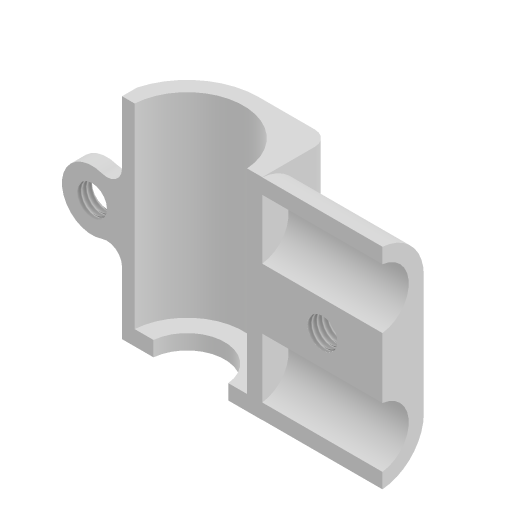
# Autodesk Inventor part: LinearBearingHolderThreaded
Saved by Autodesk Inventor 2023 (Build 270158000, 158)
## iProperties
Created: 2022-10-31
Part Number: LinearBearingHolderThreaded
Material: Generic
Document SubType Name: Modeling
Designer: deli
Density: 1 g/cm^3
Appearance: Default
Author: deli
Autodesk Inventor part; units mm, degrees
ref_plane "YZ Plane" through (0, 0, 0) normal (1, 0, 0) x (0, 1, 0)
ref_plane "XZ Plane" through (0, 0, 0) normal (0, 1, 0) x (-1, 0, 0)
ref_plane "XY Plane" through (0, 0, 0) normal (0, 0, 1) x (1, 0, 0)
sketch "Sketch2" plane through (0, 0, 0) normal (0, 1, 0) x (-1, 0, 0)
  arc A0 (14.7581, -138.6871) -> (29.7247, -138.6871) centre (22.2414, -138.1871) ccw
  line L0 (12.7414, -138.6871) -> (12.7414, -147.6871)
  arc A1 (22.2414, -147.6871) -> (31.4065, -140.6871) centre (22.2414, -138.1871) ccw
  line L1 (12.7414, -138.6871) -> (14.7581, -138.6871)
  line L2 (34.8429, -138.6871) -> (29.7247, -138.6871)
  line L3 (34.8429, -138.6871) -> (39.4065, -138.6871)
  line L4 (39.4065, -138.6871) -> (39.4065, -140.6871)
  line L5 (39.4065, -140.6871) -> (31.4065, -140.6871)
  line L6 (22.2414, -147.6871) -> (12.7414, -147.6871)
  point P0 (0, 0)
  point P1 (13.7497, -138.6871)
  dimension "d0" = 15
  dimension "d1" = 2
  dimension "d2" = 2
  dimension "d3" = 8
  dimension "d17" = 0.5
  constraints: 14 end point, 4 horizontal, 4 point on circle, 2 centre point, 2 perpendicular, 2 tangent, 1 coincident, 1 collinear, 1 midpoint, 1 vertical
  measures "d0" diameter of A0
  measures "d1" radial gap between concentric circles of A1 A0
  measures "d2" distance of L3.end L4.end
  measures "d3" distance of L4.end L5.end
  measures "d17" vertical distance of A0.centre point (13.75, -138.687)
extrude "Extrusion1" add sketch "Sketch2" along normal blind 26
sketch "Sketch3" plane through (0, 0, 0) normal (0, -1, 0) x (1, 0, 0)
  arc A0 (-31.4065, -140.6871) -> (-22.2414, -147.6871) centre (-22.2414, -138.1871) ccw projected
  line L0 (-12.7414, -147.6871) -> (-22.2414, -147.6871) projected
  line L1 (-12.7414, -138.6871) -> (-12.7414, -147.6871) projected
  line L2 (-39.4065, -140.6871) -> (-39.4065, -138.6871) projected
  line L3 (-31.4065, -140.6871) -> (-39.4065, -140.6871) projected
  line L4 (-39.4065, -138.6871) -> (-29.7247, -138.6871) projected
  arc A1 (-27.2163, -138.6871) -> (-17.2665, -138.6871) centre (-22.2414, -138.1871) ccw
  line L5 (-29.7247, -138.6871) -> (-27.2163, -138.6871)
  line L6 (-17.2665, -138.6871) -> (-12.7414, -138.6871)
  arc A2 (-29.7247, -138.6871) -> (-14.7581, -138.6871) centre (-22.2414, -138.1871) ccw construction
  point P0 (0, 0)
  dimension "d6" = 10
  constraints: 4 end point, 2 collinear, 2 point on circle, 1 centre point, 1 concentric, 1 horizontal, 1 point on line
  measures "d6" diameter of A1
extrude "Extrusion2" add sketch "Sketch3" along normal blind 2
sketch "Sketch5" plane through (-12.7414, -2, -138.6871) normal (1, 0, 0) x (0, 0, -1)
  arc A0 (0, 18.0314) -> (0, 25.9686) centre (-0.5, 22) ccw
  arc A1 (0, 2.0314) -> (0, 9.9686) centre (-0.5, 6) ccw
  arc A2 (5.5, 22) -> (0, 27.9791) centre (-0.5, 22) ccw
  arc A3 (0, 0.0209) -> (5.5, 6) centre (-0.5, 6) ccw
  line L0 (0, 28) -> (9, 28) projected
  line L1 (9, 0) -> (0, 0) projected
  line L2 (0, 0) -> (0, 28) projected
  line L3 (5.5, 22) -> (5.5, 6)
  point P0 (-138.6871, 2)
  point P1 (0, 9.9686)
  point P2 (0, 2.0314)
  point P3 (3.9152, 26)
  dimension "d18" = 8
  dimension "d19" = 2
  dimension "d20" = 0.5
  dimension "d21" = 0.5
  constraints: 8 point on circle, 6 point on line, 4 centre point, 2 coincident, 2 end point, 2 equal radius, 2 tangent, 1 vertical
  measures "d18" diameter of A0
  measures "d19" radial gap between concentric circles of A2 A0
  measures "d20" distance from line of L2 A0.centre
  measures "d21" distance from line of L2 A1.centre
extrude "Extrusion4" add sketch "Sketch5" along normal blind 16 contours A0 L2 A2 L3 A3 A1
sketch "Sketch6" plane through (-39.4065, 26, -138.6871) normal (0, 0, 1) x (1, 0, 0)
  circle A0 centre (4, -14) radius 2
  circle A1 centre (34.6652, -13.9791) radius 2
  line L0 (0, -28) -> (0, 0) projected
  line L1 (12.1902, -28) -> (0, -28) projected
  line L2 (26.6652, -27.9791) -> (42.6652, -27.9791) projected
  line L3 (26.6652, -28) -> (26.6652, 0) projected
  line L4 (42.6652, -25.9686) -> (42.6652, -27.9791) projected
  circle A2 centre (4, -14) radius 4
  line L5 (8, 1.0253) -> (8, -28)
  line L6 (0, 0) -> (9.6818, 0) projected
  arc A3 (8, -19.6569) -> (5.3333, -17.7712) centre (6, -19.6569) ccw
  arc A4 (5.3333, -10.2288) -> (8, -8.3431) centre (6, -8.3431) ccw
  point P0 (39.4065, -26)
  point P1 (26.6652, -9.9686)
  point P2 (26.6652, -2.0314)
  point P3 (42.6652, -9.9686)
  point P4 (42.6652, -20.0314)
  point P5 (8, 0)
  point P6 (0, -14)
  point P7 (8, -14)
  dimension "d22" = 4
  dimension "d24" = 4
  dimension "d25" = 14
  dimension "d26" = 28
  dimension "d27" = 14
  dimension "d28" = 16
  dimension "d29" = 8
  dimension "d32" = 4
  constraints: 6 point on circle, 6 tangent, 5 centre point, 3 point on line, 2 end point, 2 equal radius, 1 coincident, 1 vertical
  measures "d22" diameter of A0
  measures "d24" distance from line of A0.centre L0
  measures "d25" distance from line of L1 A0.centre
  measures "d26" distance of L0.start L0.end
  measures "d27" distance from line of L2 A1.centre
  measures "d28" distance between parallel lines of L3 L4
  measures "d29" distance from line of L4 A1.centre
  measures "d32" diameter of A3
extrude "Extrusion5" cut sketch "Sketch6" against normal blind 16 contours A0 | A1 | L0 A2 A3 L5 L1 | L0 L6 L5 A4 A2
thread "Thread1" size "M4x0.7" class "6H" standard "ANSI Metric M Profile" full length
thread "Thread2" size "M4x0.7" class "6H" standard "ANSI Metric M Profile" full length
fillet "Fillet1" radius 2 1 edges at (-12.7414, 12, -147.6871)
equation "\"d21\" = d20"
equation "\"d25\" = 0.5 * d26"
equation "\"d27\" = d25"
equation "\"d29\" = 0.5 * d28"
body "Solid1"
